Autodesk Fusion 360 part; units mm, degrees
note: some values were not read from the file. Set by a fixed rule: which face or edge a step refers to.
(part 2 of 2)
sketch "Sketch29" plane through (-82.5946, 0, 0) normal (-1, 0, 0) x (0, 0, 1)
  spline S0 degree 3 poles (-0.0088, 93.9597) (-0.6843, 93.1247) (-1.3301, 92.2891) (-1.9461, 91.4527) knots 0.988988 0.988988 0.988988 0.988988 1 1 1 1
  line L0 (-1.9461, 91.4527) -> (2.0923, 88.5068)
  spline S1 degree 3 poles (3.892, 90.8339) (3.2621, 90.0557) (2.6622, 89.2799) (2.0923, 88.5068) knots 0.988988 0.988988 0.988988 0.988988 1 1 1 1
  spline S2 degree 3 poles (3.892, 90.8339) (7.6038, 95.4195) (12.3442, 100.1165) (18.2038, 104.7327) (23.6789, 109.0459) (30.1513, 113.2851) (37.907, 116.9402) (41.5747, 118.6687) (45.5293, 120.2619) (49.7608, 121.6454) (53.8517, 122.9829) (58.2023, 124.124) (62.748, 124.9964) (71.4314, 126.6629) (80.8355, 127.3266) (90.1211, 126.6118) (94.5122, 126.2738) (98.8727, 125.6317) (103.1148, 124.6797) (107.216, 123.7593) (111.2058, 122.5492) (115.0262, 121.0716) (122.3241, 118.2492) (128.9869, 114.4326) (134.8901, 110.0719) (140.4059, 105.9973) (145.2707, 101.4744) (149.5279, 96.9183) (153.5058, 92.661) (156.9605, 88.3921) (159.9241, 84.1953) (162.6933, 80.2738) (165.0284, 76.4031) (166.9608, 72.3676) (168.7664, 68.5968) (170.2217, 64.6639) (171.373, 60.3743) (172.4488, 56.3661) (173.258, 52.0406) (173.8647, 47.4157) (174.9847, 38.877) (175.442, 29.3308) (175.6602, 19.7531) (175.7564, 15.5342) (175.8022, 11.3133) (175.7896, 7.1446) (175.7664, -0.5518) (175.5532, -8.0498) (174.8175, -15.405) (174.1771, -21.8068) (173.1225, -28.1278) (171.4442, -34.4461) (169.9835, -39.9454) (168.0456, -45.4489) (165.6374, -50.8308) (163.5414, -55.515) (161.0945, -60.0978) (158.3838, -64.4225) (156.0245, -68.1865) (153.4678, -71.7517) (150.7906, -75.028) (148.4604, -77.8796) (146.0401, -80.5113) (143.5749, -82.8988) (139.3355, -87.0047) (134.9708, -90.375) (130.6051, -93.1713) (127.3576, -95.2513) (124.1055, -97.0237) (120.8733, -98.5975) (116.1227, -100.9106) (111.4157, -102.8141) (106.8194, -104.4979) (102.334, -106.141) (97.9537, -107.5633) (93.697, -108.7859) knots 0 0 0 0 0.0648875 0.0648875 0.0648875 0.12551774 0.12551774 0.12551774 0.15418987 0.15418987 0.15418987 0.18190992 0.18190992 0.18190992 0.23486232 0.23486232 0.23486232 0.25990358 0.25990358 0.25990358 0.28411334 0.28411334 0.28411334 0.33036017 0.33036017 0.33036017 0.37357274 0.37357274 0.37357274 0.41395014 0.41395014 0.41395014 0.45167837 0.45167837 0.45167837 0.48693126 0.48693126 0.48693126 0.51987121 0.51987121 0.51987121 0.5806859 0.5806859 0.5806859 0.60747461 0.60747461 0.60747461 0.6569327 0.6569327 0.6569327 0.69997921 0.69997921 0.69997921 0.73744532 0.73744532 0.73744532 0.77005446 0.77005446 0.77005446 0.79843626 0.79843626 0.79843626 0.82313873 0.82313873 0.82313873 0.86562012 0.86562012 0.86562012 0.89722013 0.89722013 0.89722013 0.94366453 0.94366453 0.94366453 0.98898803 0.98898803 0.98898803 0.98898803
  line L1 (93.697, -108.7859) -> (95.1001, -113.5836)
  spline S3 degree 3 poles (-0.0088, 93.9597) (2.0055, 96.4499) (4.2822, 98.9356) (6.8298, 101.4163) (9.2928, 103.8146) (12.0084, 106.2095) (15.0068, 108.5775) (17.9056, 110.8668) (21.0705, 113.1313) (24.546, 115.3152) (27.9062, 117.4266) (31.5587, 119.4615) (35.5301, 121.3456) (39.3696, 123.1671) (43.5088, 124.847) (47.9347, 126.307) (52.2136, 127.7184) (56.7612, 128.9238) (61.5141, 129.849) (70.5934, 131.6164) (80.4339, 132.3419) (90.2111, 131.6179) (94.8348, 131.2755) (99.4396, 130.6125) (103.9326, 129.6187) (108.2763, 128.6579) (112.5147, 127.3875) (116.5778, 125.8306) (120.5059, 124.3254) (124.2694, 122.5527) (127.8304, 120.569) (134.6328, 116.7795) (140.6828, 112.2242) (145.9691, 107.4404) (150.9086, 102.9704) (155.1945, 98.3248) (158.9282, 93.7501) (162.417, 89.4756) (165.4315, 85.259) (168.0108, 80.9474) (170.4207, 76.9187) (172.4433, 72.7863) (174.0783, 68.3623) (175.606, 64.2286) (176.7916, 59.8332) (177.6917, 55.1371) (178.5328, 50.7491) (179.1291, 46.1029) (179.5641, 41.2773) (179.9706, 36.7683) (180.2385, 32.107) (180.4252, 27.3959) (180.5997, 22.9938) (180.7046, 18.5514) (180.7562, 14.1363) (180.8044, 10.0109) (180.8061, 5.9096) (180.7368, 1.8459) (180.6088, -5.6565) (180.2407, -13.0331) (179.2724, -20.3996) (178.4295, -26.811) (177.1141, -33.2309) (175.1603, -39.6404) (173.4598, -45.2191) (171.2779, -50.7859) (168.6567, -56.1806) (166.3753, -60.8759) (163.7657, -65.4349) (160.9134, -69.717) (158.4309, -73.4439) (155.7661, -76.9591) (152.9866, -80.1878) (150.5674, -82.998) (148.0618, -85.5907) (145.5116, -87.9473) (141.1259, -91.9999) (136.6133, -95.3417) (132.1322, -98.1167) (128.7989, -100.181) (125.482, -101.9405) (122.2156, -103.4995) (117.4148, -105.7909) (112.7238, -107.6688) (108.1537, -109.3321) (103.6938, -110.9553) (99.3454, -112.3637) (95.1001, -113.5836) knots 0 0 0 0 0.03284003 0.03284003 0.03284003 0.06458959 0.06458959 0.06458959 0.09528488 0.09528488 0.09528488 0.12496091 0.12496091 0.12496091 0.15365153 0.15365153 0.15365153 0.18138946 0.18138946 0.18138946 0.234376 0.234376 0.234376 0.25943342 0.25943342 0.25943342 0.28365878 0.28365878 0.28365878 0.30707973 0.30707973 0.30707973 0.35181973 0.35181973 0.35181973 0.39362435 0.39362435 0.39362435 0.43268616 0.43268616 0.43268616 0.46918512 0.46918512 0.46918512 0.50328939 0.50328939 0.50328939 0.53515608 0.53515608 0.53515608 0.564932 0.564932 0.564932 0.59275431 0.59275431 0.59275431 0.61875121 0.61875121 0.61875121 0.66674744 0.66674744 0.66674744 0.7085216 0.7085216 0.7085216 0.74488031 0.74488031 0.74488031 0.7765256 0.7765256 0.7765256 0.8040685 0.8040685 0.8040685 0.82804083 0.82804083 0.82804083 0.86926657 0.86926657 0.86926657 0.89993256 0.89993256 0.89993256 0.94500418 0.94500418 0.94500418 0.98898803 0.98898803 0.98898803 0.98898803
  spline S4 degree 5 poles (13.0954, 100.4338) (13.1864, 100.1323) (13.3793, 99.5891) (13.701, 98.9541) (14.1947, 98.4672) (14.9268, 98.4444) (15.7946, 98.9597) (16.8361, 99.9205) (18.0919, 101.2093) (19.5926, 102.6994) (21.347, 104.2711) (23.3256, 105.8312) (25.4659, 107.3149) (27.687, 108.6809) (29.9013, 109.9079) (32.0269, 110.9914) (34.0006, 111.9399) (35.7896, 112.7715) (37.4061, 113.5108) (38.8965, 114.1856) (40.3247, 114.8241) (41.7583, 115.4525) (43.2534, 116.0917) (44.8393, 116.7547) (46.5249, 117.4467) (48.3048, 118.1653) (50.1668, 118.9005) (52.0974, 119.6355) (54.0896, 120.346) (56.1415, 121.0039) (58.2521, 121.5824) (60.4181, 122.06) (62.6298, 122.4258) (64.8682, 122.6835) (67.1, 122.8573) (69.28, 122.9892) (71.3571, 123.1314) (73.2794, 123.3399) (74.9991, 123.6672) (76.4782, 124.1566) (77.6938, 124.8342) (78.447, 125.5366) (78.8873, 126.1552) (79.1255, 126.6085) (79.2308, 126.8453) knots 0 0 0 0 0 0 0.025 0.05 0.075 0.1 0.125 0.15 0.175 0.2 0.225 0.25 0.275 0.3 0.325 0.35 0.375 0.4 0.425 0.45 0.475 0.5 0.525 0.55 0.575 0.6 0.625 0.65 0.675 0.7 0.725 0.75 0.775 0.8 0.825 0.85 0.875 0.9 0.925 0.95 0.975 1 1 1 1 1 1
  line L2 (13.0954, 100.4338) -> (10.352, 104.6851)
  point P0 (14.7992, 98.5405)
  point P1 (20.2051, 103.2256)
  point P2 (34.2605, 112.0553)
  point P3 (41.8288, 115.4791)
  point P4 (50.6585, 119.083)
  point P5 (63.4525, 122.5068)
  point P6 (75.1653, 123.7681)
  constraint coincident S2 S4.start
  constraint coincident S2 S4.end
  constraint coincident S3 L2.end
extrude "Extrude1'''''''''" add sketch "Sketch29" against normal up to surface (40 mm away) separate body contours S2 S4 makes body 16 in component "Component'''''''"
sketch "Sketch30" plane through (-42.5946, 0, 0) normal (1, 0, 0) x (0, 0, -1)
  spline S0 degree 5 poles (-13.4895, -99.2308) (-13.5444, -99.0264) (-13.6695, -98.6594) (-13.9031, -98.2343) (-14.3062, -97.918) (-14.9629, -97.9205) (-15.7708, -98.2506) (-16.7266, -98.7958) (-17.8269, -99.438) (-19.0692, -100.0869) (-20.4515, -100.6995) (-21.9703, -101.2631) (-23.618, -101.7847) (-25.3813, -102.2796) (-27.238, -102.7586) (-29.1571, -103.2211) (-31.1042, -103.6603) (-33.0454, -104.0654) (-34.9519, -104.4254) (-36.8041, -104.7316) (-38.597, -104.9812) (-40.3417, -105.1789) (-42.0599, -105.333) (-43.7804, -105.4532) (-45.534, -105.5467) (-47.3495, -105.6167) (-49.2493, -105.6579) (-51.2478, -105.659) (-53.3518, -105.6067) (-55.56, -105.4884) (-57.8625, -105.2958) (-60.2407, -105.0277) (-62.6667, -104.6944) (-65.1035, -104.3187) (-67.5086, -103.9323) (-69.8366, -103.5723) (-72.0425, -103.2779) (-74.0845, -103.0867) (-75.927, -103.0318) (-77.5441, -103.1378) (-78.9211, -103.4186) (-79.8252, -103.7884) (-80.3913, -104.1482) (-80.7191, -104.4246) (-80.8706, -104.572) knots 0 0 0 0 0 0 0.025 0.05 0.075 0.1 0.125 0.15 0.175 0.2 0.225 0.25 0.275 0.3 0.325 0.35 0.375 0.4 0.425 0.45 0.475 0.5 0.525 0.55 0.575 0.6 0.625 0.65 0.675 0.7 0.725 0.75 0.775 0.8 0.825 0.85 0.875 0.9 0.925 0.95 0.975 1 1 1 1 1 1
  spline S1 degree 3 poles (-3.892, -90.8339) (-5.2727, -93.1469) (-7.6138, -95.5218) (-10.9951, -97.7495) (-14.1546, -99.831) (-18.2042, -101.7722) (-23.0866, -103.328) (-27.6487, -104.7817) (-32.9459, -105.8898) (-38.8204, -106.5134) (-44.3094, -107.0961) (-50.3044, -107.2525) (-56.5013, -107.0266) (-62.2916, -106.8156) (-68.2472, -106.2789) (-74.0547, -105.5352) (-79.4812, -104.8403) (-84.7729, -103.9696) (-89.7237, -103.0064) (-94.3497, -102.1065) (-98.6748, -101.1284) (-102.6337, -100.0784) (-106.3328, -99.0972) (-109.7138, -98.0511) (-112.8385, -96.8809) (-118.6072, -94.7205) (-123.5357, -92.1148) (-128.3713, -88.5557) (-130.5014, -86.9879) (-132.6081, -85.2388) (-134.6992, -83.3175) (-138.5597, -79.7702) (-142.3719, -75.6314) (-145.9365, -71.2127) (-149.0389, -67.3668) (-151.9404, -63.3257) (-154.4896, -59.2695) (-156.7082, -55.7391) (-158.659, -52.1965) (-160.3112, -48.6416) (-163.1525, -42.5281) (-165.1011, -36.3457) (-166.3371, -29.851) (-167.2565, -25.0199) (-167.789, -20.014) (-168.0922, -15.014) (-168.3178, -11.2947) (-168.4192, -7.5884) (-168.4662, -4.0126) (-168.5353, 1.2429) (-168.4975, 6.1962) (-168.4824, 10.608) (-168.4677, 14.9134) (-168.4682, 18.7146) (-168.5001, 21.9817) knots 0.020993 0.020993 0.020993 0.020993 0.085226 0.085226 0.085226 0.145244 0.145244 0.145244 0.201324 0.201324 0.201324 0.253726 0.253726 0.253726 0.302689 0.302689 0.302689 0.348439 0.348439 0.348439 0.391188 0.391188 0.391188 0.431132 0.431132 0.431132 0.504878 0.504878 0.504878 0.537363 0.537363 0.537363 0.597338 0.597338 0.597338 0.649538 0.649538 0.649538 0.69497 0.69497 0.69497 0.773102 0.773102 0.773102 0.831221 0.831221 0.831221 0.874453 0.874453 0.874453 0.937993 0.937993 0.937993 1 1 1 1
  line L0 (-168.5001, 21.9817) -> (-173.4727, 22.4925)
  spline S2 degree 3 poles (0.0088, -93.9597) (-1.9523, -96.9971) (-4.8952, -99.7535) (-8.7766, -102.2289) (-12.4034, -104.5419) (-16.8698, -106.6059) (-22.1423, -108.2367) (-27.0689, -109.7605) (-32.704, -110.8914) (-38.8738, -111.5118) (-44.6388, -112.0916) (-50.8684, -112.223) (-57.2559, -111.968) (-63.2244, -111.7298) (-69.3219, -111.1624) (-75.2517, -110.3885) (-80.7924, -109.6654) (-86.1807, -108.7671) (-91.2321, -107.7721) (-95.9521, -106.8424) (-100.3743, -105.8314) (-104.4627, -104.7304) (-112.0106, -102.6979) (-118.4133, -100.354) (-124.2822, -97.0861) (-126.8674, -95.6466) (-129.3542, -94.0267) (-131.7886, -92.2039) (-134.0632, -90.5006) (-136.2927, -88.6206) (-138.4875, -86.5787) (-142.5395, -82.809) (-146.4823, -78.4844) (-150.1632, -73.8814) (-153.3669, -69.875) (-156.3595, -65.6721) (-159.0015, -61.4211) (-161.301, -57.7211) (-163.3339, -53.9818) (-165.0594, -50.204) (-166.5613, -46.916) (-167.8312, -43.595) (-168.8756, -40.2237) (-170.6718, -34.4259) (-171.7915, -28.4499) (-172.4557, -22.3993) (-173.4319, -13.5063) (-173.4766, -4.5083) (-173.4706, 3.3114) (-173.4676, 7.1736) (-173.4454, 10.7507) (-173.4405, 13.9866) (-173.4357, 17.1444) (-173.4451, 19.9814) (-173.4727, 22.4925) knots 0.020993 0.020993 0.020993 0.020993 0.085226 0.085226 0.085226 0.145244 0.145244 0.145244 0.201324 0.201324 0.201324 0.253726 0.253726 0.253726 0.302689 0.302689 0.302689 0.348439 0.348439 0.348439 0.391188 0.391188 0.391188 0.470112 0.470112 0.470112 0.504878 0.504878 0.504878 0.537363 0.537363 0.537363 0.597338 0.597338 0.597338 0.649538 0.649538 0.649538 0.69497 0.69497 0.69497 0.734513 0.734513 0.734513 0.802516 0.802516 0.802516 0.902464 0.902464 0.902464 0.951828 0.951828 0.951828 1 1 1 1
  spline S3 degree 3 poles (0.0088, -93.9597) (0.6498, -92.967) (1.1841, -91.9433) (1.6056, -90.8908) knots 0 0 0 0 0.020993 0.020993 0.020993 0.020993
  line L1 (1.6056, -90.8908) -> (-2.8254, -88.577)
  spline S4 degree 3 poles (-3.892, -90.8339) (-3.4408, -90.078) (-3.0888, -89.3269) (-2.8254, -88.577) knots 0 0 0 0 0.020993 0.020993 0.020993 0.020993
  line L2 (-13.4895, -99.2308) -> (-10.4988, -103.2714)
  line L3 (-80.8706, -104.572) -> (-82.6646, -109.3056)
  point P0 (-14.6216, -97.9656)
  point P1 (-17.485, -99.2308)
  point P2 (-24.7436, -102.0943)
  point P3 (-36.1975, -104.6248)
  point P4 (-45.92, -105.5571)
  point P5 (-59.5998, -105.0908)
  point P6 (-75.4558, -103.0699)
  constraint coincident S2 L2.end
  constraint coincident S2 L3.end
extrude "Extrude1''''''''''" add sketch "Sketch30" against normal up to surface (40 mm away) contours S0 S1 L2 bodies 13 in component "Component''''''''"
component "Component" placed x (1, 0, 0) y (0, 1, 0) z (0, 0, 1) at (0, 0, 0)
component "Component'" placed x (1, 0, 0) y (0, 1, 0) z (0, 0, 1) at (0, 0, 0)
component "Component''" placed x (1, 0, 0) y (0, 1, 0) z (0, 0, 1) at (0, 0, 0)
component "Component'''" placed x (1, 0, 0) y (0, 1, 0) z (0, 0, 1) at (0, 0, 0)
component "Component''''" placed x (1, 0, 0) y (0, 1, 0) z (0, 0, 1) at (0.8533, 0, 0)
component "Component'''''" placed x (1, 0, 0) y (0, 1, 0) z (0, 0, 1) at (0, 0, 0)
component "Component''''''" placed x (1, 0, 0) y (0, 1, 0) z (0, 0, 1) at (0, 0, 0)
component "Component'''''''" placed x (1, 0, 0) y (0, 1, 0) z (0, 0, 1) at (0, 0, 0)
component "Component''''''''" placed x (1, 0, 0) y (0, 1, 0) z (0, 0, 1) at (0, 0, 0)
component "Component'''''''''" placed x (1, 0, 0) y (0, 1, 0) z (0, 0, 1) at (0, 0, 0)
